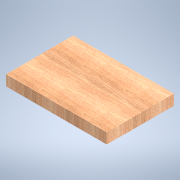
# Autodesk Inventor part: Whack01-BaseForFrisbeeShooter
Saved by Autodesk Inventor 2022 (Build 260153000, 153)
## iProperties
Created: 2021-04-23
Part Number: Whack01-BaseForFrisbeeShooter
Material: Wood (Birch)
Document SubType Name: Modeling
Designer: robst
Density: 0.55 g/cm^3
Appearance: Birch - Natural Polished
Author: robst
Autodesk Inventor part; units mm, degrees
ref_plane "YZ Plane" through (0, 0, 0) normal (1, 0, 0) x (0, 1, 0)
ref_plane "XZ Plane" through (0, 0, 0) normal (0, 1, 0) x (-1, 0, 0)
ref_plane "XY Plane" through (0, 0, 0) normal (0, 0, 1) x (1, 0, 0)
sketch "Sketch2" plane through (0, 0, 0) normal (0, 1, 0) x (-1, 0, 0)
  line L0 (304.8, 203.2) -> (-304.8, 203.2)
  line L1 (-304.8, 203.2) -> (-304.8, -203.2)
  line L2 (-304.8, -203.2) -> (304.8, -203.2)
  line L3 (304.8, -203.2) -> (304.8, 203.2)
  line L4 (304.8, 203.2) -> (-304.8, -203.2) construction
  line L5 (-304.8, 203.2) -> (304.8, -203.2) construction
  point P0 (0, 0)
  dimension "d3" = 406.4
  dimension "d4" = 609.6
  constraints: 12 end point, 2 midpoint, 2 parallel, 1 horizontal, 1 perpendicular
  measures "d3" distance of L2.end L0.start
  measures "d4" distance of L1.end L2.end
extrude "Extrusion2" add sketch "Sketch2" against normal blind 12.7
sketch "Sketch3" plane through (0, -12.7, 0) normal (0, -1, 0) x (1, 0, 0)
  line L0 (304.8, 203.2) -> (-304.8, 203.2) projected
  line L1 (304.8, -203.2) -> (304.8, 203.2) projected
  line L2 (-304.8, -203.2) -> (304.8, -203.2) projected
  line L3 (-304.8, 203.2) -> (-304.8, -203.2) projected
  line L4 (-304.8, 203.2) -> (304.8, 203.2)
  line L5 (304.8, 203.2) -> (304.8, -203.2)
  line L6 (304.8, -203.2) -> (-304.8, -203.2)
  line L7 (-304.8, -203.2) -> (-304.8, 203.2)
  line L8 (-254, 152.4) -> (-254, -152.4)
  line L9 (-254, -152.4) -> (254, -152.4)
  line L10 (254, -152.4) -> (254, 152.4)
  line L11 (254, 152.4) -> (-254, 152.4)
  line L12 (-254, 152.4) -> (254, -152.4) construction
  line L13 (-254, -152.4) -> (254, 152.4) construction
  point P0 (0, 0)
  dimension "d7" = 50.8
  dimension "d8" = 50.8
  constraints: 20 end point, 4 parallel, 2 midpoint, 2 perpendicular, 1 horizontal, 1 vertical
  measures "d7" distance between parallel lines of L3 L8
  measures "d8" distance between parallel lines of L0 L11
extrude "Extrusion3" add sketch "Sketch3" along normal blind 50.8
equation "\"d3\" = width"
equation "\"width\" = 406.4"
body "Solid2"
